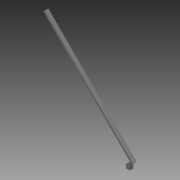
# Autodesk Inventor part: Mount
Saved by Autodesk Inventor 2013 (Build 170138000, 138)
## iProperties
Created: 2013-01-28
Part Number: Mount
Material: Generic
Document SubType Name: Modeling
Designer: Andrew Toennies
Density: 1 g/cm^3
Author: Andrew Toennies
Autodesk Inventor part; units mm, degrees
ref_plane "YZ Plane" through (0, 0, 0) normal (1, 0, 0) x (0, 1, 0)
ref_plane "XZ Plane" through (0, 0, 0) normal (0, 1, 0) x (-1, 0, 0)
ref_plane "XY Plane" through (0, 0, 0) normal (0, 0, 1) x (1, 0, 0)
sketch "Sketch1" plane through (0, 0, 0) normal (0, 0, 1) x (1, 0, 0)
  line L0 (8.9803, 8.9803) -> (-136.6846, 154.6451)
  line L1 (-136.6846, 154.6451) -> (-138.9296, 152.4)
  line L2 (-138.9296, 152.4) -> (6.7352, 6.7352)
  line L3 (6.7352, 6.7352) -> (0, 0)
  line L4 (0, 0) -> (0, -6.35)
  line L5 (0, -6.35) -> (6.35, -6.35)
  line L6 (6.35, -6.35) -> (6.35, 0)
  line L7 (6.35, 0) -> (12.1553, 5.8053)
  line L8 (8.9803, 8.9803) -> (12.1553, 5.8053)
  constraints: 18 end point, 2 vertical, 1 horizontal, 1 perpendicular, 14 other
extrude "Extrusion1" add sketch "Sketch1" along normal blind 6.35
body "Solid1"
